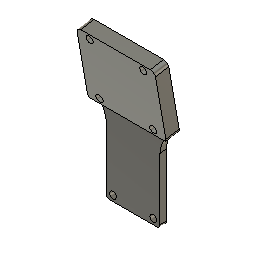
Camera Mount - Goose (Autodesk Fusion 360 design; units mm, degrees)
Autodesk Fusion 360 part; units mm, degrees
sketch "Sketch1" plane through (0, 0, 0) normal (0, 1, 0) x (1, 0, 0)
  line L0 (0, 0) -> (-12, 0) construction
  line L1 (0, 0) -> (12, 0) construction
  line L2 (-12, 0) -> (12, 0)
  line L3 (12, 0) -> (12, -40)
  line L4 (12, -40) -> (-12, -40)
  line L5 (-12, -40) -> (-12, 0)
  line L6 (0, -40) -> (0, 0) construction
  line L7 (-12, -20) -> (12, -20) construction
  line L8 (0, -2.5) -> (-9, -2.5) construction
  circle A0 centre (-9, -2.5) radius 1.5
  circle A1 centre (9, -2.5) radius 1.5
  dimension "d1" = 12
  dimension "d2" = 40
  dimension "d3" = 9
  dimension "d4" = 3
  constraint coincident L0.start L1.start
  constraint horizontal L0
  constraint parallel L0 L1
  constraint horizontal L2
  constraint vertical L3
  constraint horizontal L4
  constraint vertical L5
  constraint midpoint L4 L6.start
  constraint midpoint L3 L7.end
  constraint coincident L6 L8.start
  constraint perpendicular L6 L8
  constraint coincident L8.end A0.centre
  constraint symmetric L6 A0 A1
  measures "d1" distance of L0.start L0.end
  measures "d2" distance of L0.end L4.end
  measures "d3" distance of L8.start L8.end
  measures "d4" diameter of A0
extrude "Extrude1" add sketch "Sketch1" against normal blind 3
ref_plane "WorkPlane1" through (0, -3, 40) normal (0, -0.984808, -0.173648) x (-1, 0, 0)
sketch "Sketch2" plane through (0, 3.9309, 0.6931) normal (0, -0.984808, -0.173648) x (-1, 0, 0)
  line L0 (0, -38) -> (17.5, -38) construction
  line L1 (0.2848, -38) -> (-17.2152, -38) construction
  line L2 (17.5, -38) -> (-17.5, -38)
  line L3 (-17.5, -38) -> (-17.5, -68)
  line L4 (-17.5, -68) -> (17.5, -68)
  line L5 (17.5, -68) -> (17.5, -38)
  line L6 (0, -68) -> (0, -38) construction
  line L7 (-17.5, -53) -> (17.5, -53) construction
  line L8 (15.25, -65.65) -> (-15.25, -65.65)
  line L9 (-15.25, -65.65) -> (-15.25, -40.35)
  line L10 (-15.25, -40.35) -> (15.25, -40.35)
  line L11 (15.25, -40.35) -> (15.25, -65.65)
  line L12 (0, -65.65) -> (0, -40.35) construction
  line L13 (-15.25, -53) -> (15.25, -53) construction
  line L14 (0, -40.35) -> (12, -40.35) construction
  circle A0 centre (12, -40.35) radius 1.6
  circle A1 centre (-12, -40.35) radius 1.6
  circle A2 centre (12, -65.65) radius 1.6
  circle A3 centre (-12, -65.65) radius 1.6
  dimension "d8" = 17.5
  dimension "d9" = 17.5
  dimension "d10" = 35
  dimension "d11" = 30
  dimension "d12" = 30.5
  dimension "d13" = 25.3
  dimension "d14" = 12
  dimension "d15" = 3.2
  constraint horizontal L0
  constraint coincident L0 L1.start
  constraint parallel L0 L1
  constraint horizontal L2
  constraint vertical L3
  constraint horizontal L4
  constraint vertical L5
  constraint midpoint L4 L6.start
  constraint midpoint L3 L7.start
  constraint midpoint L5 L7.end
  constraint horizontal L8
  constraint vertical L9
  constraint horizontal L10
  constraint vertical L11
  constraint midpoint L8 L12.start
  constraint midpoint L10 L12.end
  constraint midpoint L9 L13.start
  constraint midpoint L11 L13.end
  constraint collinear L6 L12
  constraint collinear L7 L13
  constraint perpendicular L12 L14
  constraint coincident L14.end A0.centre
  constraint symmetric L6 A0 A1
  constraint symmetric L13 A0 A2
  constraint symmetric L13 A1 A3
  measures "d8" distance of L0.start L0.end
  measures "d9" distance of L1.start L1.end
  measures "d10" distance of L0.end L2.end
  measures "d11" distance of L0.end L4.end
  measures "d12" distance of L8.start L8.end
  measures "d13" distance of L8.start L10.end
  measures "d14" distance of L12.end L14.end
  measures "d15" diameter of A0
extrude "Extrude2" add sketch "Sketch2" along normal mid plane 6 contours L2 L3 L4 L5 | L8 L9 L10 L11 A0 A1 A2 A3
extrude "Extrude3" cut sketch "Sketch2" along normal mid plane 10 contours L10 A0 | L10 A0 | L10 A1 | L10 A1
fillet "Fillet1" radius 2.5 1 edges at (0, -3, 38.0572)
fillet "Fillet2" radius 10 2 edges at (12, -2.8111, 38.0905) (-12, -2.8111, 38.0905)
fillet "Fillet3" radius 2 4 edges at (-17.5, -7.8772, 67.66) (-17.5, -2.8111, 38.0905) (17.5, -7.8772, 67.66) (17.5, -2.8111, 38.0905)
fillet "Fillet4" radius 1.5 2 edges at (12, -1.5, 0) (-12, -1.5, 0)
